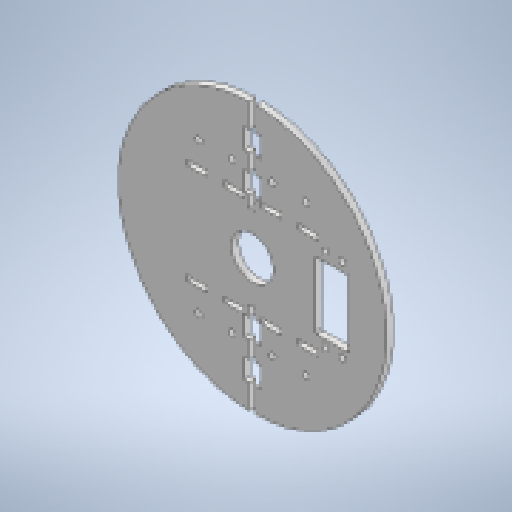
# Autodesk Inventor part: лицо1
Saved by Autodesk Inventor 2023 (Build 270158000, 158)
## iProperties
Created: 2024-12-06
Part Number: лицо1
Material: Типовые
Document SubType Name: Modeling
Designer: DELL
Density: 1 g/cm^3
Appearance: По умолчанию
Author: DELL
Autodesk Inventor part; units mm, degrees
ref_plane "YZ Plane" through (0, 0, 0) normal (1, 0, 0) x (0, 1, 0)
ref_plane "XZ Plane" through (0, 0, 0) normal (0, 1, 0) x (-1, 0, 0)
ref_plane "XY Plane" through (0, 0, 0) normal (0, 0, 1) x (1, 0, 0)
sketch "Эскиз1" plane through (0, 0, 0) normal (0, 0, 1) x (1, 0, 0)
  circle A0 centre (0, 0) radius 80 projected
  line L0 (-52.7251, -56.1362) -> (-52.7358, -38.0942) construction
  arc A1 (-51.7364, -37.0936) -> (-52.7358, -38.0942) centre (-51.7358, -38.0936) ccw construction
  line L1 (-51.7364, -37.0936) -> (-13.2571, -37.0709) construction
  arc A2 (-12.2565, -38.0703) -> (-13.2571, -37.0709) centre (-13.2565, -38.0709) ccw construction
  line L2 (-12.2565, -38.0703) -> (-12.2459, -56.1122) construction
  arc A3 (-13.2453, -57.1128) -> (-12.2459, -56.1122) centre (-13.2459, -56.1128) ccw construction
  line L3 (-13.2453, -57.1128) -> (-51.7245, -57.1356) construction
  arc A4 (-52.7251, -56.1362) -> (-51.7245, -57.1356) centre (-51.7251, -56.1356) ccw construction
  circle A5 centre (-11.4805, -27.7164) radius 3.15 construction
  circle A6 centre (-27.7164, 11.4805) radius 3.15 construction
  circle A7 centre (11.4805, 27.7164) radius 3.15 construction
  circle A8 centre (27.7164, -11.4805) radius 3.15 construction
  circle A9 centre (0, 0) radius 12.5
  circle A10 centre (0, 0) radius 39.5 construction
  point P0 (0, 0)
  dimension "d10" = 25
  constraints: 1 centre point
  measures "d10" diameter of A9
extrude "Выдавливание1" add sketch "Эскиз1" along normal blind 4
sketch "Эскиз2" plane through (0, 0, 0) normal (0, 0, -1) x (-1, 0, 0)
  circle A0 centre (0, 0) radius 80 projected
  line L0 (0, 80) -> (0, -80) construction
  line L1 (2, -80) -> (-2, -80)
  line L2 (-2, -80) -> (-2, 80)
  line L3 (-2, 80) -> (2, 80)
  line L4 (2, 80) -> (2, -80)
  line L5 (2, -80) -> (-2, 80) construction
  line L6 (-2, -80) -> (2, 80) construction
  line L7 (-2, 25) -> (2, 25)
  line L8 (-2, -25) -> (2, -25)
  point P0 (0, -25)
  point P1 (0, 80)
  point P2 (0, 25)
  dimension "d2" = 4
  dimension "d3" = 160
  dimension "d4" = 55
  dimension "d5" = 55
  constraints: 18 end point, 5 midpoint, 4 point on line, 3 perpendicular, 2 parallel, 2 point on circle, 1 horizontal, 1 vertical
  measures "d2" distance of L2.end L3.end
  measures "d3" distance of L1.end L2.end
  measures "d4" distance from line of L1 point (0, -25)
  measures "d5" distance of point (0, 80) point (0, 25)
extrude "Выдавливание2" cut sketch "Эскиз2" against normal blind 10 contours L4 L7 L2 A0 | A0 L3 L4 | L4 L1 A0 | A0 L2 L8 L4 | A0 L2 L3 | L1 L2 A0
sketch "Эскиз3" plane through (0, 0, 4) normal (0, 0, 1) x (1, 0, 0)
  line L0 (5, 53.408) -> (2, 53.408)
  line L1 (2, 31.408) -> (2, 43.408)
  line L2 (17, 28.408) -> (5, 28.408)
  line L3 (39.1243, 28.408) -> (27, 28.408)
  line L4 (2, 53.408) -> (2, 65.4106)
  line L5 (5, 65.4106) -> (5, 53.408)
  line L6 (2, 65.4106) -> (5, 65.4106)
  line L7 (2, 43.408) -> (5, 43.408)
  line L8 (5, 31.408) -> (2, 31.408)
  line L9 (5, 43.408) -> (5, 31.408)
  line L10 (5, 28.408) -> (5, 31.408)
  line L11 (5, 31.408) -> (17, 31.408)
  line L12 (27, 31.408) -> (38.9975, 31.408)
  line L13 (38.9975, 31.408) -> (39.1243, 28.408)
  line L14 (17, 31.408) -> (17, 28.408)
  line L15 (27, 28.408) -> (27, 31.408)
  line L16 (5, 65.4121) -> (5, 65.4106)
  line L17 (102, 0) -> (-112, 0) construction
  line L18 (5, -53.408) -> (2, -53.408)
  line L19 (2, -31.408) -> (2, -43.408)
  line L20 (17, -28.408) -> (5, -28.408)
  line L21 (39.1243, -28.408) -> (27, -28.408)
  line L22 (2, -53.408) -> (2, -65.4106)
  line L23 (5, -65.4106) -> (5, -53.408)
  line L24 (2, -65.4106) -> (5, -65.4106)
  line L25 (2, -43.408) -> (5, -43.408)
  line L26 (5, -31.408) -> (2, -31.408)
  line L27 (5, -43.408) -> (5, -31.408)
  line L28 (5, -28.408) -> (5, -31.408)
  line L29 (5, -31.408) -> (17, -31.408)
  line L30 (27, -31.408) -> (38.9975, -31.408)
  line L31 (38.9975, -31.408) -> (39.1243, -28.408)
  line L32 (17, -31.408) -> (17, -28.408)
  line L33 (27, -28.408) -> (27, -31.408)
  line L34 (5, -65.4121) -> (5, -65.4106)
  line L35 (0, 116) -> (0, -113) construction
  line L36 (-5, 53.408) -> (-2, 53.408)
  line L37 (-2, 31.408) -> (-2, 43.408)
  line L38 (-17, 28.408) -> (-5, 28.408)
  line L39 (-39.1243, 28.408) -> (-27, 28.408)
  line L40 (-2, 53.408) -> (-2, 65.4106)
  line L41 (-5, 65.4106) -> (-5, 53.408)
  line L42 (-2, 65.4106) -> (-5, 65.4106)
  line L43 (-2, 43.408) -> (-5, 43.408)
  line L44 (-5, 31.408) -> (-2, 31.408)
  line L45 (-5, 43.408) -> (-5, 31.408)
  line L46 (-5, 28.408) -> (-5, 31.408)
  line L47 (-5, 31.408) -> (-17, 31.408)
  line L48 (-27, 31.408) -> (-38.9975, 31.408)
  line L49 (-38.9975, 31.408) -> (-39.1243, 28.408)
  line L50 (-17, 31.408) -> (-17, 28.408)
  line L51 (-27, 28.408) -> (-27, 31.408)
  line L52 (-5, 65.4121) -> (-5, 65.4106)
  line L53 (-17, -31.408) -> (-17, -28.408)
  line L54 (-17, -28.408) -> (-5, -28.408)
  line L55 (-5, -28.408) -> (-5, -31.408)
  line L56 (-5, -31.408) -> (-17, -31.408)
  line L57 (-5, -31.408) -> (-2, -31.408)
  line L58 (-5, -43.408) -> (-5, -31.408)
  line L59 (-2, -31.408) -> (-2, -43.408)
  line L60 (-2, -43.408) -> (-5, -43.408)
  line L61 (-5, -53.408) -> (-2, -53.408)
  line L62 (-5, -65.4106) -> (-5, -53.408)
  line L63 (-5, -65.4121) -> (-5, -65.4106)
  line L64 (-2, -53.408) -> (-2, -65.4106)
  line L65 (-2, -65.4106) -> (-5, -65.4106)
  line L66 (-27, -28.408) -> (-27, -31.408)
  line L67 (-27, -31.408) -> (-38.9975, -31.408)
  line L68 (-38.9975, -31.408) -> (-39.1243, -28.408)
  line L69 (-39.1243, -28.408) -> (-27, -28.408)
  point P0 (0, 0)
  constraints: 140 end point, 48 symmetric about line, 1 horizontal, 1 vertical
extrude "Выдавливание3" cut sketch "Эскиз3" against normal blind 10
sketch "Эскиз4" plane through (0, 0, 4) normal (0, 0, 1) x (1, 0, 0)
  line L0 (39.1243, 28.408) -> (27, 28.408) projected
  line L1 (38.109, 19.5404) -> (37.0378, -18.9576) construction
  line L2 (56.5632, -20.3448) -> (37.8576, -19.8243) construction
  line L3 (56.5632, -20.3448) -> (38.109, 19.5404) construction
  line L4 (56.3361, 19.5978) -> (38.3361, 19.5978)
  line L5 (37.3361, 18.5978) -> (37.3361, -19.4022)
  line L6 (38.3361, -20.4022) -> (56.3361, -20.4022)
  line L7 (57.3361, -19.4022) -> (57.3361, 18.5978)
  line L8 (57.3361, 19.5978) -> (37.3361, -20.4022) construction
  line L9 (37.3361, 19.5978) -> (57.3361, -20.4022) construction
  arc A0 (38.3361, 19.5978) -> (37.3361, 18.5978) centre (38.3361, 18.5978) ccw
  arc A1 (37.3361, -19.4022) -> (38.3361, -20.4022) centre (38.3361, -19.4022) ccw
  arc A2 (56.3361, -20.4022) -> (57.3361, -19.4022) centre (56.3361, -19.4022) ccw
  arc A3 (57.3361, 18.5978) -> (56.3361, 19.5978) centre (56.3361, 18.5978) ccw
  point P0 (0, 0)
  point P1 (47.3361, -0.4022)
  dimension "d33" = 20
  dimension "d34" = 40
  dimension "d35" = 1
  constraints: 14 end point, 8 point on circle, 8 point on line, 8 tangent, 4 centre point, 3 equal radius, 3 midpoint, 2 parallel, 1 horizontal, 1 perpendicular
  measures "d33" distance of L9.end L8.end
  measures "d34" distance of L8.end L9.start
  measures "d35" radius of A0
extrude "Выдавливание4" cut sketch "Эскиз4" against normal blind 10
sketch "Эскиз6" plane through (0, 0, 4) normal (0, 0, 1) x (1, 0, 0)
  circle A0 centre (43.4545, -24.8018) radius 1.95
  circle A1 centre (53.4545, -24.8018) radius 1.95
  line L0 (43.4545, -24.8018) -> (53.4545, -24.8018) construction
  line L1 (53.4545, -24.8018) -> (53.4545, 24.9376) construction
  line L2 (53.4545, 24.9376) -> (43.4545, 24.9376) construction
  line L3 (43.4545, 24.9376) -> (43.4545, -24.8018) construction
  line L4 (43.4545, -24.8018) -> (53.4545, 24.9376) construction
  circle A2 centre (43.4545, 24.9376) radius 1.95
  circle A3 centre (53.4545, 24.9376) radius 1.95
  point P0 (0, 0)
  point P1 (48.4545, 0.0679)
  dimension "d15" = 3.9
  dimension "d16" = 49.7394
  dimension "d17" = 10
  dimension "d18" = 48.4545
  dimension "d20" = 3.9
  dimension "d21" = 3.9
  dimension "d22" = 3.9
  constraints: 10 end point, 4 centre point, 3 perpendicular, 2 coincident, 1 horizontal, 1 midpoint
  measures "d15" diameter of A0
  measures "d16" distance of L0.end L1.end
  measures "d17" distance of L1.end L2.end
  measures "d18" distance of point (0, 0) point (48.454, 0.068)
  measures "d20" diameter of A2
  measures "d21" diameter of A3
  measures "d22" diameter of A1
extrude "Выдавливание5" cut sketch "Эскиз6" against normal blind 10
sketch "Эскиз8" plane through (0, 0, 4) normal (0, 0, 1) x (1, 0, 0)
  circle A0 centre (-32, 44.908) radius 2.55 construction
  circle A1 centre (-12, 44.908) radius 2.55 construction
  circle A2 centre (12, 44.908) radius 2.55 construction
  circle A3 centre (32, 44.908) radius 2.55 construction
  circle A4 centre (32, -44.908) radius 2.55 construction
  circle A5 centre (12, -44.908) radius 2.55 construction
  circle A6 centre (-32, -44.908) radius 2.55 construction
  circle A7 centre (-12, -44.908) radius 2.55 construction
  circle A8 centre (-32, 44.908) radius 1.95
  circle A9 centre (-12, 44.908) radius 1.95
  circle A10 centre (12, 44.908) radius 1.95
  circle A11 centre (32, 44.908) radius 1.95
  circle A12 centre (-32, -44.908) radius 1.95
  circle A13 centre (-12, -44.908) radius 1.95
  circle A14 centre (12, -44.908) radius 1.95
  circle A15 centre (32, -44.908) radius 1.95
  point P0 (0, 0)
  dimension "d23" = 3.9
  dimension "d24" = 3.9
  dimension "d25" = 3.9
  dimension "d26" = 3.9
  dimension "d27" = 3.9
  dimension "d28" = 3.9
  dimension "d29" = 3.9
  dimension "d30" = 3.9
  constraints: 8 centre point, 8 coincident
  measures "d23" diameter of A8
  measures "d24" diameter of A9
  measures "d25" diameter of A10
  measures "d26" diameter of A11
  measures "d27" diameter of A12
  measures "d28" diameter of A13
  measures "d29" diameter of A14
  measures "d30" diameter of A15
extrude "Выдавливание6" cut sketch "Эскиз8" against normal blind 10
